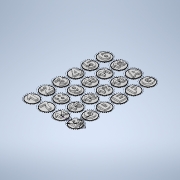
# Autodesk Inventor part: labels
Saved by Autodesk Inventor 2021 (Build 250183000, 183)
## iProperties
Created: 2023-10-09
Part Number: labels
Material: Generic
Document SubType Name: Modeling
Designer: assman
Density: 1 g/cm^3
Appearance: Default
Author: assman
Autodesk Inventor part; units mm, degrees
ref_plane "YZ Plane" through (0, 0, 0) normal (1, 0, 0) x (0, 1, 0)
ref_plane "XZ Plane" through (0, 0, 0) normal (0, 1, 0) x (-1, 0, 0)
ref_plane "XY Plane" through (0, 0, 0) normal (0, 0, 1) x (1, 0, 0)
sketch "Sketch1" plane through (0, 0, 0) normal (0, 1, 0) x (-1, 0, 0)
  circle A0 centre (0, 0) radius 6.35 construction
  circle A1 centre (0, 0) radius 5.35
  line L0 (0, 0) -> (0, -40.2986) construction
  line L1 (0, 0) -> (18.5903, 0) construction
  circle A2 centre (13, 0) radius 5.35
  circle A3 centre (13, 0) radius 6.35 construction
  circle A4 centre (26, 0) radius 5.35
  circle A5 centre (26, 0) radius 6.35 construction
  circle A6 centre (39, 0) radius 5.35
  circle A7 centre (39, 0) radius 6.35 construction
  circle A8 centre (0, -13) radius 5.35
  circle A9 centre (0, -13) radius 6.35 construction
  circle A10 centre (13, -13) radius 5.35
  circle A11 centre (13, -13) radius 6.35 construction
  circle A12 centre (26, -13) radius 5.35
  circle A13 centre (26, -13) radius 6.35 construction
  circle A14 centre (39, -13) radius 5.35
  circle A15 centre (39, -13) radius 6.35 construction
  circle A16 centre (0, -26) radius 5.35
  circle A17 centre (0, -26) radius 6.35 construction
  circle A18 centre (13, -26) radius 5.35
  circle A19 centre (13, -26) radius 6.35 construction
  circle A20 centre (26, -26) radius 5.35
  circle A21 centre (26, -26) radius 6.35 construction
  circle A22 centre (39, -26) radius 5.35
  circle A23 centre (39, -26) radius 6.35 construction
  circle A24 centre (0, -39) radius 5.35
  circle A25 centre (0, -39) radius 6.35 construction
  circle A26 centre (13, -39) radius 5.35
  circle A27 centre (13, -39) radius 6.35 construction
  circle A28 centre (26, -39) radius 5.35
  circle A29 centre (26, -39) radius 6.35 construction
  circle A30 centre (39, -39) radius 5.35
  circle A31 centre (39, -39) radius 6.35 construction
  circle A32 centre (0, -52) radius 5.35
  circle A33 centre (0, -52) radius 6.35 construction
  circle A34 centre (13, -52) radius 5.35
  circle A35 centre (13, -52) radius 6.35 construction
  circle A36 centre (26, -52) radius 5.35
  circle A37 centre (26, -52) radius 6.35 construction
  circle A38 centre (39, -52) radius 5.35
  circle A39 centre (39, -52) radius 6.35 construction
  circle A40 centre (0, -65) radius 5.35
  circle A41 centre (0, -65) radius 6.35 construction
  circle A42 centre (13, -65) radius 5.35
  circle A43 centre (13, -65) radius 6.35 construction
  circle A44 centre (26, -65) radius 5.35
  circle A45 centre (26, -65) radius 6.35 construction
  circle A46 centre (39, -65) radius 5.35
  circle A47 centre (39, -65) radius 6.35 construction
  line L2 (-5.0267, 0.6574) -> (13.5636, 0.6574) construction
  line L3 (42.8941, -1.691) -> (35.1059, -1.691)
  line L4 (35.1059, -1.691) -> (35.1059, 0.4605)
  line L5 (35.1059, 0.4605) -> (40.2121, 0.4605)
  spline S0 degree 2 poles (40.2121, 0.4605) (39.8142, 0.9837) (39.3279, 1.9562) (39.0995, 2.6931) knots 0 0 0 1 2 2 2
  line L6 (39.0995, 2.6931) -> (40.8457, 2.6931)
  spline S1 degree 2 poles (40.8457, 2.6931) (41.192, 1.6099) (42.172, 0.4089) (42.8941, 0.07) knots 0 0 0 1 2 2 2
  line L7 (42.8941, 0.07) -> (42.8941, -1.691)
  line L8 (35.1059, -16.0909) -> (35.1059, -9.7101)
  spline S2 degree 2 poles (35.1059, -9.7101) (36.049, -9.8206) (37.7143, -10.9332) (38.849, -12.4658) knots 0 0 0 1 2 2 2
  spline S3 degree 2 poles (38.849, -12.4658) (39.5416, -13.3942) (40.2636, -13.9173) (40.5878, -13.9173) knots 0 0 0 1 2 2 2
  spline S4 degree 2 poles (40.5878, -13.9173) (40.9415, -13.9173) (41.4352, -13.4016) (41.4352, -13.0111) knots 0 0 0 1 2 2 2
  spline S5 degree 2 poles (41.4352, -13.0111) (41.4352, -12.5984) (40.9268, -12.0827) (40.2784, -11.9942) knots 0 0 0 1 2 2 2
  line L9 (40.2784, -11.9942) -> (40.4478, -9.8648)
  spline S6 degree 2 poles (40.4478, -9.8648) (41.3468, -9.9901) (42.3562, -10.6606) (42.8941, -11.8764) (42.8941, -12.9521) knots 0 0 0 1 2 3 3 3
  spline S7 degree 2 poles (42.8941, -12.9521) (42.8941, -14.0721) (42.3783, -15.3247) (41.3247, -16.0394) (40.6615, -16.0394) knots 0 0 0 1 2 3 3 3
  spline S8 degree 2 poles (40.6615, -16.0394) (39.9615, -16.0394) (38.6869, -15.2215) (37.9206, -14.1384) knots 0 0 0 1 2 2 2
  spline S9 degree 2 poles (37.9206, -14.1384) (37.4785, -13.4974) (37.1248, -13.0626) (36.8374, -12.7679) knots 0 0 0 1 2 2 2
  line L10 (36.8374, -12.7679) -> (36.8374, -16.0909)
  line L11 (36.8374, -16.0909) -> (35.1059, -16.0909)
  line L12 (40.6173, -24.9353) -> (40.9784, -22.9238)
  spline S10 degree 2 poles (40.9784, -22.9238) (41.9362, -23.1743) (42.9604, -24.5964) (42.9604, -25.9005) knots 0 0 0 1 2 2 2
  spline S11 degree 2 poles (42.9604, -25.9005) (42.9604, -27.4036) (41.8404, -28.7373) (41.0005, -28.7373) knots 0 0 0 1 2 2 2
  spline S12 degree 2 poles (41.0005, -28.7373) (40.4994, -28.7373) (39.6963, -28.192) (39.3942, -27.6394) knots 0 0 0 1 2 2 2
  spline S13 degree 2 poles (39.3942, -27.6394) (39.2837, -28.0889) (39.1363, -28.3247) knots 0 0 0 1 1 1
  spline S14 degree 2 poles (39.1363, -28.3247) (38.9005, -28.7078) (38.1342, -29.1278) (37.6037, -29.1278) knots 0 0 0 1 2 2 2
  spline S15 degree 2 poles (37.6037, -29.1278) (36.9332, -29.1278) (35.7027, -28.4278) (35.0396, -27.1163) (35.0396, -26.0405) knots 0 0 0 1 2 3 3 3
  spline S16 degree 2 poles (35.0396, -26.0405) (35.0396, -25.0016) (35.5333, -23.7932) (36.4764, -23.0122) (37.1911, -22.8059) knots 0 0 0 1 2 3 3 3
  line L13 (37.1911, -22.8059) -> (37.4711, -24.9353)
  spline S17 degree 2 poles (37.4711, -24.9353) (36.8301, -25.0606) (36.3364, -25.5837) (36.3364, -25.9889) knots 0 0 0 1 2 2 2
  spline S18 degree 2 poles (36.3364, -25.9889) (36.3364, -26.4163) (36.9627, -26.9837) (37.4858, -26.9837) knots 0 0 0 1 2 2 2
  spline S19 degree 2 poles (37.4858, -26.9837) (38.0237, -26.9837) (38.6058, -26.4384) (38.6058, -25.9668) knots 0 0 0 1 2 2 2
  spline S20 degree 2 poles (38.6058, -25.9668) (38.6058, -25.7163) (38.4805, -25.2816) knots 0 0 0 1 1 1
  line L14 (38.4805, -25.2816) -> (40.0058, -25.3921)
  spline S21 degree 2 poles (40.0058, -25.3921) (39.9763, -25.569) (39.9763, -25.6647) knots 0 0 0 1 1 1
  spline S22 degree 2 poles (39.9763, -25.6647) (39.9763, -26.0847) (40.5068, -26.6447) (40.8752, -26.6447) knots 0 0 0 1 2 2 2
  spline S23 degree 2 poles (40.8752, -26.6447) (41.2215, -26.6447) (41.6415, -26.2247) (41.6415, -25.8637) knots 0 0 0 1 2 2 2
  spline S24 degree 2 poles (41.6415, -25.8637) (41.6415, -25.4879) (41.1847, -25.0163) (40.6173, -24.9353) knots 0 0 0 1 2 2 2
  line L15 (36.5353, -39.5268) -> (36.5353, -35.6512)
  line L16 (36.5353, -35.6512) -> (38.289, -35.6512)
  line L17 (38.289, -35.6512) -> (42.8941, -39.5268)
  line L18 (42.8941, -39.5268) -> (42.8941, -41.3836)
  line L19 (42.8941, -41.3836) -> (38.1858, -41.3836)
  line L20 (38.1858, -41.3836) -> (38.1858, -42.3415)
  line L21 (38.1858, -42.3415) -> (36.5353, -42.3415)
  line L22 (36.5353, -42.3415) -> (36.5353, -41.3836)
  line L23 (36.5353, -41.3836) -> (35.1059, -41.3836)
  line L24 (35.1059, -41.3836) -> (35.1059, -39.5268)
  line L25 (35.1059, -39.5268) -> (36.5353, -39.5268)
  line L26 (38.1858, -39.5268) -> (40.6026, -39.5268)
  line L27 (40.6026, -39.5268) -> (38.1858, -37.4785)
  line L28 (38.1858, -37.4785) -> (38.1858, -39.5268)
  line L29 (42.8941, -49.7343) -> (42.8941, -54.7741)
  line L30 (42.8941, -54.7741) -> (41.1994, -54.7741)
  line L31 (41.1994, -54.7741) -> (41.1994, -51.3627)
  line L32 (41.1994, -51.3627) -> (40.05, -51.1858)
  spline S25 degree 2 poles (40.05, -51.1858) (40.2121, -51.5395) (40.3815, -52.2321) (40.3815, -52.571) knots 0 0 0 1 2 2 2
  spline S26 degree 2 poles (40.3815, -52.571) (40.3815, -53.7131) (38.9889, -55.1425) (37.9353, -55.1425) knots 0 0 0 1 2 2 2
  spline S27 degree 2 poles (37.9353, -55.1425) (37.1985, -55.1425) (35.828, -54.4057) (35.1059, -53.0573) (35.1059, -52.0037) knots 0 0 0 1 2 3 3 3
  spline S28 degree 2 poles (35.1059, -52.0037) (35.1059, -51.2448) (35.3933, -50.169) (35.9606, -49.4101) (36.6827, -48.9385) (37.2206, -48.7838) knots 0 0 0 1 2 3 4 4 4
  line L33 (37.2206, -48.7838) -> (37.4564, -50.9353)
  spline S29 degree 2 poles (37.4564, -50.9353) (36.9406, -51.0163) (36.4027, -51.5837) (36.4027, -51.9816) knots 0 0 0 1 2 2 2
  spline S30 degree 2 poles (36.4027, -51.9816) (36.4027, -52.4237) (37.0732, -52.9984) (37.7437, -52.9984) knots 0 0 0 1 2 2 2
  spline S31 degree 2 poles (37.7437, -52.9984) (38.429, -52.9984) (39.0626, -52.4163) (39.0626, -51.9374) knots 0 0 0 1 2 2 2
  spline S32 degree 2 poles (39.0626, -51.9374) (39.0626, -51.6279) (38.9079, -51.3405) knots 0 0 0 1 1 1
  spline S33 degree 2 poles (38.9079, -51.3405) (38.8047, -51.1342) (38.5174, -50.8764) knots 0 0 0 1 1 1
  line L34 (38.5174, -50.8764) -> (38.7753, -49.0638)
  line L35 (38.7753, -49.0638) -> (42.8941, -49.7343)
  line L36 (41.1036, -68.0246) -> (40.8457, -65.91)
  spline S34 degree 2 poles (40.8457, -65.91) (41.2878, -65.8289) (41.6562, -65.4384) (41.6562, -65.151) knots 0 0 0 1 2 2 2
  spline S35 degree 2 poles (41.6562, -65.151) (41.6562, -64.6353) (41.1331, -64.3479) knots 0 0 0 1 1 1
  spline S36 degree 2 poles (41.1331, -64.3479) (40.7573, -64.1342) (39.5195, -64.0385) knots 0 0 0 1 1 1
  spline S37 degree 2 poles (39.5195, -64.0385) (39.91, -64.4216) (40.2784, -65.2247) (40.2784, -65.7479) knots 0 0 0 1 2 2 2
  spline S38 degree 2 poles (40.2784, -65.7479) (40.2784, -66.772) (38.8195, -68.1867) (37.6922, -68.1867) knots 0 0 0 1 2 2 2
  spline S39 degree 2 poles (37.6922, -68.1867) (36.9332, -68.1867) (35.6806, -67.472) (35.0396, -66.2047) (35.0396, -65.2468) knots 0 0 0 1 2 3 3 3
  spline S40 degree 2 poles (35.0396, -65.2468) (35.0396, -64.0974) (35.8206, -62.7122) (37.5448, -61.8796) (38.9595, -61.8796) knots 0 0 0 1 2 3 3 3
  spline S41 degree 2 poles (38.9595, -61.8796) (41.0299, -61.8796) (42.9604, -63.6258) (42.9604, -65.1658) knots 0 0 0 1 2 2 2
  spline S42 degree 2 poles (42.9604, -65.1658) (42.9604, -66.0794) (42.5404, -67.1405) (41.7225, -67.8404) (41.1036, -68.0246) knots 0 0 0 1 2 3 3 3
  spline S43 degree 2 poles (37.6922, -64.1121) (37.0732, -64.1121) (36.3659, -64.7384) (36.3659, -65.1879) knots 0 0 0 1 2 2 2
  spline S44 degree 2 poles (36.3659, -65.1879) (36.3659, -65.6079) (36.9995, -66.1679) (37.6332, -66.1679) knots 0 0 0 1 2 2 2
  spline S45 degree 2 poles (37.6332, -66.1679) (38.2816, -66.1679) (38.9595, -65.5858) (38.9595, -65.151) knots 0 0 0 1 2 2 2
  spline S46 degree 2 poles (38.9595, -65.151) (38.9595, -64.709) (38.3037, -64.1121) (37.6922, -64.1121) knots 0 0 0 1 2 2 2
  line L37 (28.628, -63.7532) -> (23.46, -63.7532)
  line L38 (23.46, -63.7532) -> (23.46, -62.3255)
  line L39 (23.46, -62.3255) -> (26.8483, -62.3255)
  spline S47 degree 2 poles (26.8483, -62.3255) (26.5843, -61.9784) (26.2616, -61.333) (26.11, -60.8441) knots 0 0 0 1 2 2 2
  line L40 (26.11, -60.8441) -> (27.2688, -60.8441)
  spline S48 degree 2 poles (27.2688, -60.8441) (27.4986, -61.5628) (28.1489, -62.3598) (28.628, -62.5847) knots 0 0 0 1 2 2 2
  line L41 (28.628, -62.5847) -> (28.628, -63.7532)
  line L42 (27.0732, -66.6624) -> (27.3128, -65.3276)
  spline S49 degree 2 poles (27.3128, -65.3276) (27.9484, -65.4938) (28.628, -66.4375) (28.628, -67.3029) knots 0 0 0 1 2 2 2
  spline S50 degree 2 poles (28.628, -67.3029) (28.628, -68.3003) (27.8848, -69.1853) (27.3274, -69.1853) knots 0 0 0 1 2 2 2
  spline S51 degree 2 poles (27.3274, -69.1853) (26.995, -69.1853) (26.462, -68.8234) (26.2616, -68.4567) knots 0 0 0 1 2 2 2
  spline S52 degree 2 poles (26.2616, -68.4567) (26.1882, -68.755) (26.0905, -68.9115) knots 0 0 0 1 1 1
  spline S53 degree 2 poles (26.0905, -68.9115) (25.934, -69.1657) (25.4255, -69.4444) (25.0735, -69.4444) knots 0 0 0 1 2 2 2
  spline S54 degree 2 poles (25.0735, -69.4444) (24.6285, -69.4444) (23.812, -68.9799) (23.372, -68.1096) (23.372, -67.3958) knots 0 0 0 1 2 3 3 3
  spline S55 degree 2 poles (23.372, -67.3958) (23.372, -66.7064) (23.6996, -65.9045) (24.3254, -65.3863) (24.7997, -65.2494) knots 0 0 0 1 2 3 3 3
  line L43 (24.7997, -65.2494) -> (24.9855, -66.6624)
  spline S56 degree 2 poles (24.9855, -66.6624) (24.5601, -66.7455) (24.2325, -67.0926) (24.2325, -67.3615) knots 0 0 0 1 2 2 2
  spline S57 degree 2 poles (24.2325, -67.3615) (24.2325, -67.6451) (24.6481, -68.0216) (24.9952, -68.0216) knots 0 0 0 1 2 2 2
  spline S58 degree 2 poles (24.9952, -68.0216) (25.3522, -68.0216) (25.7384, -67.6598) (25.7384, -67.3469) knots 0 0 0 1 2 2 2
  spline S59 degree 2 poles (25.7384, -67.3469) (25.7384, -67.1806) (25.6553, -66.8922) knots 0 0 0 1 1 1
  line L44 (25.6553, -66.8922) -> (26.6674, -66.9655)
  spline S60 degree 2 poles (26.6674, -66.9655) (26.6478, -67.0828) (26.6478, -67.1464) knots 0 0 0 1 1 1
  spline S61 degree 2 poles (26.6478, -67.1464) (26.6478, -67.4251) (26.9999, -67.7967) (27.2443, -67.7967) knots 0 0 0 1 2 2 2
  spline S62 degree 2 poles (27.2443, -67.7967) (27.4741, -67.7967) (27.7528, -67.518) (27.7528, -67.2784) knots 0 0 0 1 2 2 2
  spline S63 degree 2 poles (27.7528, -67.2784) (27.7528, -67.0291) (27.4497, -66.7162) (27.0732, -66.6624) knots 0 0 0 1 2 2 2
  line L45 (28.584, -50.7532) -> (23.416, -50.7532)
  line L46 (23.416, -50.7532) -> (23.416, -49.3255)
  line L47 (23.416, -49.3255) -> (26.8043, -49.3255)
  spline S64 degree 2 poles (26.8043, -49.3255) (26.5403, -48.9784) (26.2176, -48.333) (26.066, -47.8441) knots 0 0 0 1 2 2 2
  line L48 (26.066, -47.8441) -> (27.2248, -47.8441)
  spline S65 degree 2 poles (27.2248, -47.8441) (27.4546, -48.5628) (28.1049, -49.3598) (28.584, -49.5847) knots 0 0 0 1 2 2 2
  line L49 (28.584, -49.5847) -> (28.584, -50.7532)
  line L50 (28.584, -55.491) -> (23.416, -55.491)
  line L51 (23.416, -55.491) -> (23.416, -54.0633)
  line L52 (23.416, -54.0633) -> (26.8043, -54.0633)
  spline S66 degree 2 poles (26.8043, -54.0633) (26.5403, -53.7162) (26.2176, -53.0708) (26.066, -52.5818) knots 0 0 0 1 2 2 2
  line L53 (26.066, -52.5818) -> (27.2248, -52.5818)
  spline S67 degree 2 poles (27.2248, -52.5818) (27.4546, -53.3006) (28.1049, -54.0975) (28.584, -54.3224) knots 0 0 0 1 2 2 2
  line L54 (28.584, -54.3224) -> (28.584, -55.491)
  line L55 (28.628, -37.7532) -> (23.46, -37.7532)
  line L56 (23.46, -37.7532) -> (23.46, -36.3255)
  line L57 (23.46, -36.3255) -> (26.8483, -36.3255)
  spline S68 degree 2 poles (26.8483, -36.3255) (26.5843, -35.9784) (26.2616, -35.333) (26.11, -34.8441) knots 0 0 0 1 2 2 2
  line L58 (26.11, -34.8441) -> (27.2688, -34.8441)
  spline S69 degree 2 poles (27.2688, -34.8441) (27.4986, -35.5628) (28.1489, -36.3598) (28.628, -36.5847) knots 0 0 0 1 2 2 2
  line L59 (28.628, -36.5847) -> (28.628, -37.7532)
  spline S70 degree 2 poles (26.022, -39.2934) (27.4692, -39.2934) (28.628, -40.3348) (28.628, -41.4007) knots 0 0 0 1 2 2 2
  spline S71 degree 2 poles (28.628, -41.4007) (28.628, -41.914) (28.3738, -42.5692) (27.968, -42.9848) (27.523, -43.2244) (27.2248, -43.2977) knots 0 0 0 1 2 3 4 4 4
  spline S72 degree 2 poles (27.2248, -43.2977) (26.6576, -43.4395) (26.0367, -43.4395) knots 0 0 0 1 1 1
  spline S73 degree 2 poles (26.0367, -43.4395) (24.653, -43.4395) (23.372, -42.5056) (23.372, -41.3615) knots 0 0 0 1 2 2 2
  spline S74 degree 2 poles (23.372, -41.3615) (23.372, -40.721) (23.7827, -39.9339) (24.1787, -39.6796) knots 0 0 0 1 2 2 2
  spline S75 degree 2 poles (24.1787, -39.6796) (24.4574, -39.4987) (25.4304, -39.2934) (26.022, -39.2934) knots 0 0 0 1 2 2 2
  spline S76 degree 2 poles (26.0171, -40.6917) (25.0441, -40.6917) (24.3352, -41.034) (24.3352, -41.3567) knots 0 0 0 1 2 2 2
  spline S77 degree 2 poles (24.3352, -41.3567) (24.3352, -41.5718) (24.6383, -41.8896) (25.2886, -42.0363) (25.978, -42.0363) knots 0 0 0 1 2 3 3 3
  spline S78 degree 2 poles (25.978, -42.0363) (26.9901, -42.0363) (27.6893, -41.694) (27.6893, -41.3518) knots 0 0 0 1 2 2 2
  spline S79 degree 2 poles (27.6893, -41.3518) (27.6893, -41.0046) (26.9803, -40.6917) (26.0171, -40.6917) knots 0 0 0 1 2 2 2
  line L60 (23.889, -22.9606) -> (24.1543, -25.0753)
  spline S80 degree 2 poles (24.1543, -25.0753) (23.7122, -25.1563) (23.3438, -25.5542) (23.3438, -25.8416) knots 0 0 0 1 2 2 2
  spline S81 degree 2 poles (23.3438, -25.8416) (23.3438, -26.3574) (23.8595, -26.6447) knots 0 0 0 1 1 1
  spline S82 degree 2 poles (23.8595, -26.6447) (24.2427, -26.851) (25.4805, -26.9542) knots 0 0 0 1 1 1
  spline S83 degree 2 poles (25.4805, -26.9542) (25.09, -26.571) (24.7216, -25.7679) (24.7216, -25.2448) knots 0 0 0 1 2 2 2
  spline S84 degree 2 poles (24.7216, -25.2448) (24.7216, -24.2132) (26.1805, -22.7985) (27.3005, -22.7985) knots 0 0 0 1 2 2 2
  spline S85 degree 2 poles (27.3005, -22.7985) (28.0668, -22.7985) (29.3194, -23.5206) (29.9604, -24.7806) (29.9604, -25.7384) knots 0 0 0 1 2 3 3 3
  spline S86 degree 2 poles (29.9604, -25.7384) (29.9604, -26.8879) (29.172, -28.2731) (27.4552, -29.1057) (26.0405, -29.1057) knots 0 0 0 1 2 3 3 3
  spline S87 degree 2 poles (26.0405, -29.1057) (23.9701, -29.1057) (22.0396, -27.3594) (22.0396, -25.8195) knots 0 0 0 1 2 2 2
  spline S88 degree 2 poles (22.0396, -25.8195) (22.0396, -24.9058) (22.4596, -23.8448) (23.2775, -23.1522) (23.889, -22.9606) knots 0 0 0 1 2 3 3 3
  spline S89 degree 2 poles (27.3078, -26.8731) (27.9268, -26.8731) (28.6341, -26.2468) (28.6341, -25.7974) knots 0 0 0 1 2 2 2
  spline S90 degree 2 poles (28.6341, -25.7974) (28.6341, -25.3774) (28.0005, -24.8174) (27.3594, -24.8174) knots 0 0 0 1 2 2 2
  spline S91 degree 2 poles (27.3594, -24.8174) (26.7184, -24.8174) (26.0405, -25.3995) (26.0405, -25.8342) knots 0 0 0 1 2 2 2
  spline S92 degree 2 poles (26.0405, -25.8342) (26.0405, -26.2837) (26.6963, -26.8731) (27.3078, -26.8731) knots 0 0 0 1 2 2 2
  spline S93 degree 2 poles (26.2837, -11.1543) (26.5489, -10.6532) (26.8805, -10.4248) knots 0 0 0 1 1 1
  spline S94 degree 2 poles (26.8805, -10.4248) (27.33, -10.108) (27.912, -10.108) knots 0 0 0 1 1 1
  spline S95 degree 2 poles (27.912, -10.108) (28.8773, -10.108) (29.4888, -11.0069) knots 0 0 0 1 1 1
  spline S96 degree 2 poles (29.4888, -11.0069) (29.9604, -11.7143) (29.9604, -12.8711) knots 0 0 0 1 1 1
  spline S97 degree 2 poles (29.9604, -12.8711) (29.9604, -14.4036) (28.7889, -15.8699) (27.8973, -15.8699) knots 0 0 0 1 2 2 2
  spline S98 degree 2 poles (27.8973, -15.8699) (27.3815, -15.8699) (26.9321, -15.5752) knots 0 0 0 1 1 1
  spline S99 degree 2 poles (26.9321, -15.5752) (26.5931, -15.3615) (26.2837, -14.8899) knots 0 0 0 1 1 1
  spline S100 degree 2 poles (26.2837, -14.8899) (25.9816, -15.5089) (25.0016, -16.1204) (24.4048, -16.1204) knots 0 0 0 1 2 2 2
  spline S101 degree 2 poles (24.4048, -16.1204) (23.8374, -16.1204) (22.8354, -15.5973) (22.2975, -14.8236) (22.0396, -13.6816) (22.0396, -13.0405) knots 0 0 0 1 2 3 4 4 4
  spline S102 degree 2 poles (22.0396, -13.0405) (22.0396, -11.8248) (22.6143, -10.5427) (23.7269, -9.8722) (24.4195, -9.8722) knots 0 0 0 1 2 3 3 3
  spline S103 degree 2 poles (24.4195, -9.8722) (25.09, -9.8722) (26.0258, -10.4985) (26.2837, -11.1543) knots 0 0 0 1 2 2 2
  spline S104 degree 2 poles (24.4932, -11.9942) (23.9848, -11.9942) (23.3438, -12.6058) (23.3438, -13.0037) knots 0 0 0 1 2 2 2
  spline S105 degree 2 poles (23.3438, -13.0037) (23.3438, -13.3795) (23.9995, -13.9837) (24.5006, -13.9837) knots 0 0 0 1 2 2 2
  spline S106 degree 2 poles (24.5006, -13.9837) (25.0016, -13.9837) (25.65, -13.3795) (25.65, -12.9742) knots 0 0 0 1 2 2 2
  spline S107 degree 2 poles (25.65, -12.9742) (25.65, -12.5837) (25.0237, -11.9942) (24.4932, -11.9942) knots 0 0 0 1 2 2 2
  spline S108 degree 2 poles (27.7868, -12.1121) (27.3889, -12.1121) (26.9026, -12.6058) (26.9026, -13.0111) knots 0 0 0 1 2 2 2
  spline S109 degree 2 poles (26.9026, -13.0111) (26.9026, -13.3795) (27.3815, -13.8437) (27.7647, -13.8437) knots 0 0 0 1 2 2 2
  spline S110 degree 2 poles (27.7647, -13.8437) (28.1626, -13.8437) (28.6636, -13.3574) (28.6636, -12.9816) knots 0 0 0 1 2 2 2
  spline S111 degree 2 poles (28.6636, -12.9816) (28.6636, -12.5911) (28.1773, -12.1121) (27.7868, -12.1121) knots 0 0 0 1 2 2 2
  line L61 (29.8278, 3.0909) -> (29.8278, -3.1131)
  line L62 (29.8278, -3.1131) -> (28.391, -3.1131)
  spline S112 degree 2 poles (28.391, -3.1131) (27.6615, -2.3026) (26.8068, -1.7647) knots 0 0 0 1 1 1
  spline S113 degree 2 poles (26.8068, -1.7647) (25.7753, -1.1089) (24.5079, -0.7258) knots 0 0 0 1 1 1
  spline S114 degree 2 poles (24.5079, -0.7258) (23.5206, -0.4237) (22.1722, -0.3205) knots 0 0 0 1 1 1
  line L63 (22.1722, -0.3205) -> (22.1722, 1.8015)
  spline S115 degree 2 poles (22.1722, 1.8015) (24.0438, 1.551) (26.5858, 0.4752) (28.0299, -0.6889) knots 0 0 0 1 2 2 2
  line L64 (28.0299, -0.6889) -> (28.0299, 3.0909)
  line L65 (28.0299, 3.0909) -> (29.8278, 3.0909)
  line L66 (15.584, 1.2468) -> (10.416, 1.2468)
  line L67 (10.416, 1.2468) -> (10.416, 2.6745)
  line L68 (10.416, 2.6745) -> (13.8043, 2.6745)
  spline S116 degree 2 poles (13.8043, 2.6745) (13.5403, 3.0216) (13.2176, 3.667) (13.066, 4.1559) knots 0 0 0 1 2 2 2
  line L69 (13.066, 4.1559) -> (14.2248, 4.1559)
  spline S117 degree 2 poles (14.2248, 4.1559) (14.4546, 3.4372) (15.1049, 2.6402) (15.584, 2.4153) knots 0 0 0 1 2 2 2
  line L70 (15.584, 2.4153) -> (15.584, 1.2468)
  line L71 (11.3645, -2.7185) -> (11.3645, -0.1467)
  line L72 (11.3645, -0.1467) -> (12.5282, -0.1467)
  line L73 (12.5282, -0.1467) -> (15.584, -2.7185)
  line L74 (15.584, -2.7185) -> (15.584, -3.9506)
  line L75 (15.584, -3.9506) -> (12.4597, -3.9506)
  line L76 (12.4597, -3.9506) -> (12.4597, -4.5862)
  line L77 (12.4597, -4.5862) -> (11.3645, -4.5862)
  line L78 (11.3645, -4.5862) -> (11.3645, -3.9506)
  line L79 (11.3645, -3.9506) -> (10.416, -3.9506)
  line L80 (10.416, -3.9506) -> (10.416, -2.7185)
  line L81 (10.416, -2.7185) -> (11.3645, -2.7185)
  line L82 (12.4597, -2.7185) -> (14.0634, -2.7185)
  line L83 (14.0634, -2.7185) -> (12.4597, -1.3592)
  line L84 (12.4597, -1.3592) -> (12.4597, -2.7185)
  line L85 (15.628, -11.7532) -> (10.46, -11.7532)
  line L86 (10.46, -11.7532) -> (10.46, -10.3255)
  line L87 (10.46, -10.3255) -> (13.8483, -10.3255)
  spline S118 degree 2 poles (13.8483, -10.3255) (13.5843, -9.9784) (13.2616, -9.333) (13.11, -8.8441) knots 0 0 0 1 2 2 2
  line L88 (13.11, -8.8441) -> (14.2688, -8.8441)
  spline S119 degree 2 poles (14.2688, -8.8441) (14.4986, -9.5628) (15.1489, -10.3598) (15.628, -10.5847) knots 0 0 0 1 2 2 2
  line L89 (15.628, -10.5847) -> (15.628, -11.7532)
  line L90 (15.54, -13.8654) -> (15.54, -17.2097)
  line L91 (15.54, -17.2097) -> (14.4155, -17.2097)
  line L92 (14.4155, -17.2097) -> (14.4155, -14.9459)
  line L93 (14.4155, -14.9459) -> (13.6527, -14.8286)
  spline S120 degree 2 poles (13.6527, -14.8286) (13.7603, -15.0633) (13.8727, -15.5229) (13.8727, -15.7478) knots 0 0 0 1 2 2 2
  spline S121 degree 2 poles (13.8727, -15.7478) (13.8727, -16.5056) (12.9487, -17.4542) (12.2495, -17.4542) knots 0 0 0 1 2 2 2
  spline S122 degree 2 poles (12.2495, -17.4542) (11.7606, -17.4542) (10.8511, -16.9652) (10.372, -16.0705) (10.372, -15.3713) knots 0 0 0 1 2 3 3 3
  spline S123 degree 2 poles (10.372, -15.3713) (10.372, -14.8677) (10.5627, -14.1539) (10.9392, -13.6503) (11.4183, -13.3374) (11.7752, -13.2347) knots 0 0 0 1 2 3 4 4 4
  line L94 (11.7752, -13.2347) -> (11.9317, -14.6624)
  spline S124 degree 2 poles (11.9317, -14.6624) (11.5894, -14.7162) (11.2325, -15.0926) (11.2325, -15.3567) knots 0 0 0 1 2 2 2
  spline S125 degree 2 poles (11.2325, -15.3567) (11.2325, -15.65) (11.6774, -16.0314) (12.1224, -16.0314) knots 0 0 0 1 2 2 2
  spline S126 degree 2 poles (12.1224, -16.0314) (12.5771, -16.0314) (12.9976, -15.6451) (12.9976, -15.3273) knots 0 0 0 1 2 2 2
  spline S127 degree 2 poles (12.9976, -15.3273) (12.9976, -15.122) (12.8949, -14.9313) knots 0 0 0 1 1 1
  spline S128 degree 2 poles (12.8949, -14.9313) (12.8264, -14.7944) (12.6357, -14.6233) knots 0 0 0 1 1 1
  line L95 (12.6357, -14.6233) -> (12.8069, -13.4205)
  line L96 (12.8069, -13.4205) -> (15.54, -13.8654)
  line L97 (15.628, -24.7532) -> (10.46, -24.7532)
  line L98 (10.46, -24.7532) -> (10.46, -23.3255)
  line L99 (10.46, -23.3255) -> (13.8483, -23.3255)
  spline S129 degree 2 poles (13.8483, -23.3255) (13.5843, -22.9784) (13.2616, -22.333) (13.11, -21.8441) knots 0 0 0 1 2 2 2
  line L100 (13.11, -21.8441) -> (14.2688, -21.8441)
  spline S130 degree 2 poles (14.2688, -21.8441) (14.4986, -22.5628) (15.1489, -23.3598) (15.628, -23.5847) knots 0 0 0 1 2 2 2
  line L101 (15.628, -23.5847) -> (15.628, -24.7532)
  line L102 (14.3959, -30.3759) -> (14.2248, -28.9727)
  spline S131 degree 2 poles (14.2248, -28.9727) (14.5181, -28.9189) (14.7626, -28.6598) (14.7626, -28.4691) knots 0 0 0 1 2 2 2
  spline S132 degree 2 poles (14.7626, -28.4691) (14.7626, -28.1269) (14.4155, -27.9362) knots 0 0 0 1 1 1
  spline S133 degree 2 poles (14.4155, -27.9362) (14.1661, -27.7944) (13.3447, -27.7308) knots 0 0 0 1 1 1
  spline S134 degree 2 poles (13.3447, -27.7308) (13.6038, -27.9851) (13.8483, -28.518) (13.8483, -28.8651) knots 0 0 0 1 2 2 2
  spline S135 degree 2 poles (13.8483, -28.8651) (13.8483, -29.5448) (12.8802, -30.4835) (12.1321, -30.4835) knots 0 0 0 1 2 2 2
  spline S136 degree 2 poles (12.1321, -30.4835) (11.6285, -30.4835) (10.7974, -30.0092) (10.372, -29.1683) (10.372, -28.5327) knots 0 0 0 1 2 3 3 3
  spline S137 degree 2 poles (10.372, -28.5327) (10.372, -27.7699) (10.8903, -26.8507) (12.0344, -26.2982) (12.9731, -26.2982) knots 0 0 0 1 2 3 3 3
  spline S138 degree 2 poles (12.9731, -26.2982) (14.347, -26.2982) (15.628, -27.457) (15.628, -28.4789) knots 0 0 0 1 2 2 2
  spline S139 degree 2 poles (15.628, -28.4789) (15.628, -29.0852) (15.3493, -29.7892) (14.8066, -30.2537) (14.3959, -30.3759) knots 0 0 0 1 2 3 3 3
  spline S140 degree 2 poles (12.1321, -27.7797) (11.7214, -27.7797) (11.2521, -28.1953) (11.2521, -28.4936) knots 0 0 0 1 2 2 2
  spline S141 degree 2 poles (11.2521, -28.4936) (11.2521, -28.7722) (11.6726, -29.1438) (12.093, -29.1438) knots 0 0 0 1 2 2 2
  spline S142 degree 2 poles (12.093, -29.1438) (12.5233, -29.1438) (12.9731, -28.7576) (12.9731, -28.4691) knots 0 0 0 1 2 2 2
  spline S143 degree 2 poles (12.9731, -28.4691) (12.9731, -28.1757) (12.538, -27.7797) (12.1321, -27.7797) knots 0 0 0 1 2 2 2
  line L103 (15.584, -37.7532) -> (10.416, -37.7532)
  line L104 (10.416, -37.7532) -> (10.416, -36.3255)
  line L105 (10.416, -36.3255) -> (13.8043, -36.3255)
  spline S144 degree 2 poles (13.8043, -36.3255) (13.5403, -35.9784) (13.2176, -35.333) (13.066, -34.8441) knots 0 0 0 1 2 2 2
  line L106 (13.066, -34.8441) -> (14.2248, -34.8441)
  spline S145 degree 2 poles (14.2248, -34.8441) (14.4546, -35.5628) (15.1049, -36.3598) (15.584, -36.5847) knots 0 0 0 1 2 2 2
  line L107 (15.584, -36.5847) -> (15.584, -37.7532)
  line L108 (15.496, -39.3178) -> (15.496, -43.4346)
  line L109 (15.496, -43.4346) -> (14.5426, -43.4346)
  spline S146 degree 2 poles (14.5426, -43.4346) (14.0585, -42.8968) (13.4914, -42.5399) knots 0 0 0 1 1 1
  spline S147 degree 2 poles (13.4914, -42.5399) (12.8069, -42.1047) (11.9659, -41.8505) knots 0 0 0 1 1 1
  spline S148 degree 2 poles (11.9659, -41.8505) (11.3107, -41.65) (10.416, -41.5816) knots 0 0 0 1 1 1
  line L110 (10.416, -41.5816) -> (10.416, -40.1734)
  spline S149 degree 2 poles (10.416, -40.1734) (11.6579, -40.3397) (13.3447, -41.0535) (14.303, -41.826) knots 0 0 0 1 2 2 2
  line L111 (14.303, -41.826) -> (14.303, -39.3178)
  line L112 (14.303, -39.3178) -> (15.496, -39.3178)
  line L113 (15.628, -50.7532) -> (10.46, -50.7532)
  line L114 (10.46, -50.7532) -> (10.46, -49.3255)
  line L115 (10.46, -49.3255) -> (13.8483, -49.3255)
  spline S150 degree 2 poles (13.8483, -49.3255) (13.5843, -48.9784) (13.2616, -48.333) (13.11, -47.8441) knots 0 0 0 1 2 2 2
  line L116 (13.11, -47.8441) -> (14.2688, -47.8441)
  spline S151 degree 2 poles (14.2688, -47.8441) (14.4986, -48.5628) (15.1489, -49.3598) (15.628, -49.5847) knots 0 0 0 1 2 2 2
  line L117 (15.628, -49.5847) -> (15.628, -50.7532)
  spline S152 degree 2 poles (13.1882, -53.1441) (13.3643, -52.8116) (13.5843, -52.6601) knots 0 0 0 1 1 1
  spline S153 degree 2 poles (13.5843, -52.6601) (13.8825, -52.4498) (14.2688, -52.4498) knots 0 0 0 1 1 1
  spline S154 degree 2 poles (14.2688, -52.4498) (14.9093, -52.4498) (15.3151, -53.0463) knots 0 0 0 1 1 1
  spline S155 degree 2 poles (15.3151, -53.0463) (15.628, -53.5157) (15.628, -54.2833) knots 0 0 0 1 1 1
  spline S156 degree 2 poles (15.628, -54.2833) (15.628, -55.3003) (14.8506, -56.2733) (14.259, -56.2733) knots 0 0 0 1 2 2 2
  spline S157 degree 2 poles (14.259, -56.2733) (13.9167, -56.2733) (13.6185, -56.0777) knots 0 0 0 1 1 1
  spline S158 degree 2 poles (13.6185, -56.0777) (13.3936, -55.9359) (13.1882, -55.623) knots 0 0 0 1 1 1
  spline S159 degree 2 poles (13.1882, -55.623) (12.9878, -56.0337) (12.3375, -56.4395) (11.9415, -56.4395) knots 0 0 0 1 2 2 2
  spline S160 degree 2 poles (11.9415, -56.4395) (11.565, -56.4395) (10.9, -56.0924) (10.5431, -55.579) (10.372, -54.8211) (10.372, -54.3958) knots 0 0 0 1 2 3 4 4 4
  spline S161 degree 2 poles (10.372, -54.3958) (10.372, -53.589) (10.7534, -52.7383) (11.4916, -52.2934) (11.9512, -52.2934) knots 0 0 0 1 2 3 3 3
  spline S162 degree 2 poles (11.9512, -52.2934) (12.3962, -52.2934) (13.0171, -52.709) (13.1882, -53.1441) knots 0 0 0 1 2 2 2
  spline S163 degree 2 poles (12.0001, -53.7015) (11.6628, -53.7015) (11.2374, -54.1073) (11.2374, -54.3713) knots 0 0 0 1 2 2 2
  spline S164 degree 2 poles (11.2374, -54.3713) (11.2374, -54.6207) (11.6726, -55.0216) (12.005, -55.0216) knots 0 0 0 1 2 2 2
  spline S165 degree 2 poles (12.005, -55.0216) (12.3375, -55.0216) (12.7678, -54.6207) (12.7678, -54.3518) knots 0 0 0 1 2 2 2
  spline S166 degree 2 poles (12.7678, -54.3518) (12.7678, -54.0926) (12.3522, -53.7015) (12.0001, -53.7015) knots 0 0 0 1 2 2 2
  spline S167 degree 2 poles (14.1857, -53.7797) (13.9216, -53.7797) (13.5989, -54.1073) (13.5989, -54.3762) knots 0 0 0 1 2 2 2
  spline S168 degree 2 poles (13.5989, -54.3762) (13.5989, -54.6207) (13.9167, -54.9287) (14.171, -54.9287) knots 0 0 0 1 2 2 2
  spline S169 degree 2 poles (14.171, -54.9287) (14.435, -54.9287) (14.7675, -54.606) (14.7675, -54.3567) knots 0 0 0 1 2 2 2
  spline S170 degree 2 poles (14.7675, -54.3567) (14.7675, -54.0975) (14.4448, -53.7797) (14.1857, -53.7797) knots 0 0 0 1 2 2 2
  line L118 (10.7063, -66.1815) -> (10.7063, -63.7723)
  line L119 (10.7063, -63.7723) -> (9.571, -63.4357)
  line L120 (9.571, -63.4357) -> (9.571, -61.2707)
  line L121 (9.571, -61.2707) -> (16.429, -63.8515)
  line L122 (16.429, -63.8515) -> (16.429, -66.1683)
  line L123 (16.429, -66.1683) -> (9.571, -68.7425)
  line L124 (9.571, -68.7425) -> (9.571, -66.5247)
  line L125 (9.571, -66.5247) -> (10.7063, -66.1815)
  line L126 (12.1914, -65.7393) -> (14.6534, -64.9868)
  line L127 (14.6534, -64.9868) -> (12.1914, -64.2343)
  line L128 (12.1914, -64.2343) -> (12.1914, -65.7393)
  line L129 (-0.9823, -65.1711) -> (0.4963, -65.1711)
  line L130 (0.4963, -65.1711) -> (0.4963, -68.5663)
  line L131 (0.4963, -68.5663) -> (-2.5292, -68.5663)
  spline S171 degree 2 poles (-2.5292, -68.5663) (-3.2001, -67.5874) (-3.6792, -66.0884) (-3.6792, -65.0616) knots 0 0 0 1 2 2 2
  spline S172 degree 2 poles (-3.6792, -65.0616) (-3.6792, -63.7953) (-2.8167, -62.1935) (-1.1055, -61.3174) (0.0034, -61.3174) knots 0 0 0 1 2 3 3 3
  spline S173 degree 2 poles (0.0034, -61.3174) (1.1671, -61.3174) (2.8852, -62.2757) (3.337, -63.2066) knots 0 0 0 1 2 2 2
  spline S174 degree 2 poles (3.337, -63.2066) (3.6792, -63.9322) (3.6792, -65.1506) knots 0 0 0 1 1 1
  spline S175 degree 2 poles (3.6792, -65.1506) (3.6792, -66.3348) (3.2548, -67.5053) (2.3513, -68.2788) (1.6668, -68.4704) knots 0 0 0 1 2 3 3 3
  line L132 (1.6668, -68.4704) -> (1.2834, -66.3485)
  spline S176 degree 2 poles (1.2834, -66.3485) (1.6873, -66.2184) (2.1185, -65.5887) (2.1185, -65.1027) knots 0 0 0 1 2 2 2
  spline S177 degree 2 poles (2.1185, -65.1027) (2.1185, -64.3839) (1.1123, -63.5215) (0.024, -63.5215) knots 0 0 0 1 2 2 2
  spline S178 degree 2 poles (0.024, -63.5215) (-1.126, -63.5215) (-2.1185, -64.3908) (-2.1185, -65.1711) knots 0 0 0 1 2 2 2
  spline S179 degree 2 poles (-2.1185, -65.1711) (-2.1185, -65.5408) (-1.9063, -66.2116) (-1.6462, -66.6428) knots 0 0 0 1 2 2 2
  line L133 (-1.6462, -66.6428) -> (-0.9823, -66.6428)
  line L134 (-0.9823, -66.6428) -> (-0.9823, -65.1711)
  line L135 (3.556, -49.4228) -> (3.556, -54.851)
  line L136 (3.556, -54.851) -> (2.0296, -54.851)
  line L137 (2.0296, -54.851) -> (2.0296, -51.6338)
  line L138 (2.0296, -51.6338) -> (0.7906, -51.6338)
  line L139 (0.7906, -51.6338) -> (0.7906, -54.3787)
  line L140 (0.7906, -54.3787) -> (-0.6469, -54.3787)
  line L141 (-0.6469, -54.3787) -> (-0.6469, -51.6338)
  line L142 (-0.6469, -51.6338) -> (-3.556, -51.6338)
  line L143 (-3.556, -51.6338) -> (-3.556, -49.4228)
  line L144 (-3.556, -49.4228) -> (3.556, -49.4228)
  line L145 (3.556, -36.1353) -> (3.556, -42.0221)
  line L146 (3.556, -42.0221) -> (2.0364, -42.0221)
  line L147 (2.0364, -42.0221) -> (2.0364, -38.3395)
  line L148 (2.0364, -38.3395) -> (0.907, -38.3395)
  line L149 (0.907, -38.3395) -> (0.907, -41.7551)
  line L150 (0.907, -41.7551) -> (-0.5442, -41.7551)
  line L151 (-0.5442, -41.7551) -> (-0.5442, -38.3395)
  line L152 (-0.5442, -38.3395) -> (-1.9474, -38.3395)
  line L153 (-1.9474, -38.3395) -> (-1.9474, -42.1316)
  line L154 (-1.9474, -42.1316) -> (-3.556, -42.1316)
  line L155 (-3.556, -42.1316) -> (-3.556, -36.1353)
  line L156 (-3.556, -36.1353) -> (3.556, -36.1353)
  line L157 (3.556, -22.8924) -> (3.556, -26.1574)
  spline S180 degree 2 poles (3.556, -26.1574) (3.556, -27.1226) (3.0289, -28.3136) (2.0501, -29.0871) (0.7495, -29.4362) (0.024, -29.4362) knots 0 0 0 1 2 3 4 4 4
  spline S181 degree 2 poles (0.024, -29.4362) (-1.1192, -29.4362) (-2.3718, -28.916) (-3.2206, -27.9988) (-3.3643, -27.4648) knots 0 0 0 1 2 3 3 3
  spline S182 degree 2 poles (-3.3643, -27.4648) (-3.556, -26.7461) (-3.556, -26.1574) knots 0 0 0 1 1 1
  line L158 (-3.556, -26.1574) -> (-3.556, -22.8924)
  line L159 (-3.556, -22.8924) -> (3.556, -22.8924)
  line L160 (1.9474, -25.0896) -> (-1.9406, -25.0896)
  line L161 (-1.9406, -25.0896) -> (-1.9406, -25.6304)
  spline S183 degree 2 poles (-1.9406, -25.6304) (-1.9406, -26.3149) (-1.6325, -26.8967) (-0.8727, -27.2253) (-0.0171, -27.2253) knots 0 0 0 1 2 3 3 3
  spline S184 degree 2 poles (-0.0171, -27.2253) (1.1123, -27.2253) (1.9474, -26.486) (1.9474, -25.6372) knots 0 0 0 1 2 2 2
  line L162 (1.9474, -25.6372) -> (1.9474, -25.0896)
  line L163 (-0.6469, -14.5949) -> (-1.2287, -16.5184)
  spline S185 degree 2 poles (-1.2287, -16.5184) (-2.0364, -16.3267) (-3.1248, -15.4916) (-3.6792, -14.2526) (-3.6792, -13.3012) knots 0 0 0 1 2 3 3 3
  spline S186 degree 2 poles (-3.6792, -13.3012) (-3.6792, -12.1375) (-3.0016, -10.6727) (-1.304, -9.6049) (0.0171, -9.6049) knots 0 0 0 1 2 3 3 3
  spline S187 degree 2 poles (0.0171, -9.6049) (1.7831, -9.6049) (3.6792, -11.4804) (3.6792, -13.1985) knots 0 0 0 1 2 2 2
  spline S188 degree 2 poles (3.6792, -13.1985) (3.6792, -14.5401) (2.5908, -16.0734) (1.4683, -16.4499) knots 0 0 0 1 2 2 2
  line L164 (1.4683, -16.4499) -> (1.037, -14.5059)
  spline S189 degree 2 poles (1.037, -14.5059) (1.3587, -14.4032) (1.5093, -14.2937) knots 0 0 0 1 1 1
  spline S190 degree 2 poles (1.5093, -14.2937) (1.7626, -14.1089) (2.0364, -13.575) (2.0364, -13.2464) knots 0 0 0 1 2 2 2
  spline S191 degree 2 poles (2.0364, -13.2464) (2.0364, -12.5072) (1.434, -12.1101) knots 0 0 0 1 1 1
  spline S192 degree 2 poles (1.434, -12.1101) (0.9891, -11.809) (0.0308, -11.809) knots 0 0 0 1 1 1
  spline S193 degree 2 poles (0.0308, -11.809) (-1.1534, -11.809) (-2.0296, -12.5277) (-2.0296, -13.178) knots 0 0 0 1 2 2 2
  spline S194 degree 2 poles (-2.0296, -13.178) (-2.0296, -13.8077) (-1.3245, -14.4511) (-0.6469, -14.5949) knots 0 0 0 1 2 2 2
  line L165 (3.556, 3.135) -> (3.556, -0.9788)
  spline S195 degree 2 poles (3.556, -0.9788) (3.556, -2.0056) (2.5361, -3.1076) (1.7831, -3.1076) knots 0 0 0 1 2 2 2
  spline S196 degree 2 poles (1.7831, -3.1076) (1.1534, -3.1076) (0.7016, -2.7175) knots 0 0 0 1 1 1
  spline S197 degree 2 poles (0.7016, -2.7175) (0.4004, -2.4505) (0.2225, -1.944) knots 0 0 0 1 1 1
  spline S198 degree 2 poles (0.2225, -1.944) (0.0376, -2.7106) (-0.8591, -3.4362) (-1.5367, -3.4362) knots 0 0 0 1 2 2 2
  spline S199 degree 2 poles (-1.5367, -3.4362) (-2.0843, -3.4362) (-2.9673, -2.9228) (-3.2274, -2.4779) knots 0 0 0 1 2 2 2
  spline S200 degree 2 poles (-3.2274, -2.4779) (-3.3849, -2.1973) (-3.4602, -1.6428) knots 0 0 0 1 1 1
  spline S201 degree 2 poles (-3.4602, -1.6428) (-3.556, -0.8967) (-3.556, -0.6571) knots 0 0 0 1 1 1
  line L166 (-3.556, -0.6571) -> (-3.556, 3.135)
  line L167 (-3.556, 3.135) -> (3.556, 3.135)
  line L168 (-2.0296, 0.9172) -> (-2.0296, -0.1985)
  spline S202 degree 2 poles (-2.0296, -0.1985) (-2.0296, -0.7666) (-1.6257, -1.2321) (-1.2903, -1.2321) knots 0 0 0 1 2 2 2
  spline S203 degree 2 poles (-1.2903, -1.2321) (-0.9754, -1.2321) (-0.5921, -0.7735) (-0.5921, -0.1985) knots 0 0 0 1 2 2 2
  line L169 (-0.5921, -0.1985) -> (-0.5921, 0.9172)
  line L170 (-0.5921, 0.9172) -> (-2.0296, 0.9172)
  line L171 (0.7632, 0.9172) -> (0.7632, -0.0342)
  spline S204 degree 2 poles (0.7632, -0.0342) (0.7632, -0.5476) (1.1192, -0.9515) (1.4546, -0.9515) knots 0 0 0 1 2 2 2
  spline S205 degree 2 poles (1.4546, -0.9515) (1.7626, -0.9515) (2.1117, -0.5476) (2.1117, -0.0479) knots 0 0 0 1 2 2 2
  line L172 (2.1117, -0.0479) -> (2.1117, 0.9172)
  line L173 (2.1117, 0.9172) -> (0.7632, 0.9172)
  line L174 (42.8941, -1.691) -> (35.1059, -1.691)
  line L175 (35.1059, -1.691) -> (35.1059, 0.4605)
  line L176 (35.1059, 0.4605) -> (40.2121, 0.4605)
  spline S206 degree 2 poles (40.2121, 0.4605) (39.8142, 0.9837) (39.3279, 1.9562) (39.0995, 2.6931) knots 0 0 0 1 2 2 2
  line L177 (39.0995, 2.6931) -> (40.8457, 2.6931)
  spline S207 degree 2 poles (40.8457, 2.6931) (41.192, 1.6099) (42.172, 0.4089) (42.8941, 0.07) knots 0 0 0 1 2 2 2
  line L178 (42.8941, 0.07) -> (42.8941, -1.691)
  point P0 (13, -13)
  point P1 (13, -26)
  point P2 (13, -39)
  point P3 (0, -13)
  point P4 (0, -26)
  point P5 (0, -39)
  point P6 (0, -52)
  point P7 (0, -65)
  point P8 (13, -52)
  point P9 (13, -65)
  dimension "d0" = 12.7
  dimension "d1" = 1
  dimension "d4" = 13
  dimension "d7" = 13
  constraints: 48 centre point, 25 coincident, 6 end point, 3 horizontal, 2 vertical, 93 other
  measures "d0" diameter of A0
  measures "d1" radial gap between concentric circles of A0 A1
  measures "d4" distance of L0.start A2.centre
  measures "d7" distance of L0.start A8.centre
extrude "Extrusion1" add sketch "Sketch1" along normal blind 1.2 contours L3 L4 L5 S0 L6 S1 L7 | L8 S2 S3 S4 S5 L9 S6 S7 S8 S9 L10 L11 | L12 S10 S11 S12 S13 S14 S15 S16 L13 S17 S18 S19 S20 L14 S21 S22 S23 S24 | L15 L16 L17 L18 L19 L20 L21 L22 L23 L24 L25 | L29 L30 L31 L32 S25 S26 S27 S28 L33 S29 S30 S31 S32 S33 L34 L35 | L36 S34 S35 S36 S37 S38 S39 S40 S41 S42 | L37 L38 L39 S47 L40 S48 L41 | L42 S49 S50 S51 S52 S53 S54 S55 L43 S56 S57 S58 S59 L44 S60 S61 S62 S63 | L45 L46 L47 S64 L48 S65 L49 | L50 L51 L52 S66 L53 S67 L54 | L55 L56 L57 S68 L58 S69 L59 | S70 S71 S72 S73 S74 S75 | L60 S80 S81 S82 S83 S84 S85 S86 S87 S88 | S93 S94 S95 S96 S97 S98 S99 S100 S101 S102 S103 | L61 L62 S112 S113 S114 L63 S115 L64 L65 | L66 L67 L68 S116 L69 S117 L70 | L71 L72 L73 L74 L75 L76 L77 L78 L79 L80 L81 | L85 L86 L87 S118 L88 S119 L89 | L90 L91 L92 L93 S120 S121 S122 S123 L94 S124 S125 S126 S127 S128 L95 L96 | L97 L98 L99 S129 L100 S130 L101 | L102 S131 S132 S133 S134 S135 S136 S137 S138 S139 | L103 L104 L105 S144 L106 S145 L107 | L108 L109 S146 S147 S148 L110 S149 L111 L112 | L113 L114 L115 S150 L116 S151 L117 | S152 S153 S154 S155 S156 S157 S158 S159 S160 S161 S162 | L118 L119 L120 L121 L122 L123 L124 L125 | L129 L130 L131 S171 S172 S173 S174 S175 L132 S176 S177 S178 S179 L133 L134 | L135 L136 L137 L138 L139 L140 L141 L142 L143 L144 | L145 L146 L147 L148 L149 L150 L151 L152 L153 L154 L155 L156 | L157 S180 S181 S182 L158 L159 | L163 S185 S186 S187 S188 L164 S189 S190 S191 S192 S193 S194 | L165 S195 S196 S197 S198 S199 S200 S201 L166 L167
extrude "Extrusion2" add sketch "Sketch1" against normal blind 0.8 contours A1 | A2 | A4 | A6 | A8 | A10 | A12 | A14 | A16 | A18 | A20 | A22 | A24 | A26 | A28 | A30 | A32 | A34 | A36 | A38 | A40 | A42 | A44 | A46 | L3 L4 L5 S0 L6 S1 L7 | L8 S2 S3 S4 S5 L9 S6 S7 S8 S9 L10 L11 | L12 S10 S11 S12 S13 S14 S15 S16 L13 S17 S18 S19 S20 L14 S21 S22 S23 S24 | L15 L16 L17 L18 L19 L20 L21 L22 L23 L24 L25 | L28 L27 L26 | L29 L30 L31 L32 S25 S26 S27 S28 L33 S29 S30 S31 S32 S33 L34 L35 | L36 S34 S35 S36 S37 S38 S39 S40 S41 S42 | S46 S45 S44 S43 | L37 L38 L39 S47 L40 S48 L41 | L42 S49 S50 S51 S52 S53 S54 S55 L43 S56 S57 S58 S59 L44 S60 S61 S62 S63 | L45 L46 L47 S64 L48 S65 L49 | L50 L51 L52 S66 L53 S67 L54 | L55 L56 L57 S68 L58 S69 L59 | S70 S71 S72 S73 S74 S75 | S79 S78 S77 S76 | L60 S80 S81 S82 S83 S84 S85 S86 S87 S88 | S92 S91 S90 S89 | S93 S94 S95 S96 S97 S98 S99 S100 S101 S102 S103 | S107 S106 S105 S104 | S111 S110 S109 S108 | L61 L62 S112 S113 S114 L63 S115 L64 L65 | L66 L67 L68 S116 L69 S117 L70 | L71 L72 L73 L74 L75 L76 L77 L78 L79 L80 L81 | L84 L83 L82 | L85 L86 L87 S118 L88 S119 L89 | L90 L91 L92 L93 S120 S121 S122 S123 L94 S124 S125 S126 S127 S128 L95 L96 | L97 L98 L99 S129 L100 S130 L101 | L102 S131 S132 S133 S134 S135 S136 S137 S138 S139 | S143 S142 S141 S140 | L103 L104 L105 S144 L106 S145 L107 | L108 L109 S146 S147 S148 L110 S149 L111 L112 | L113 L114 L115 S150 L116 S151 L117 | S152 S153 S154 S155 S156 S157 S158 S159 S160 S161 S162 | S166 S165 S164 S163 | S170 S169 S168 S167 | L118 L119 L120 L121 L122 L123 L124 L125 | L128 L127 L126 | L129 L130 L131 S171 S172 S173 S174 S175 L132 S176 S177 S178 S179 L133 L134 | L135 L136 L137 L138 L139 L140 L141 L142 L143 L144 | L145 L146 L147 L148 L149 L150 L151 L152 L153 L154 L155 L156 | L157 S180 S181 S182 L158 L159 | L162 S184 S183 L161 L160 | L163 S185 S186 S187 S188 L164 S189 S190 S191 S192 S193 S194 | L165 S195 S196 S197 S198 S199 S200 S201 L166 L167 | L170 L169 S203 S202 L168 | L173 L172 S205 S204 L171
body "Solid1"
